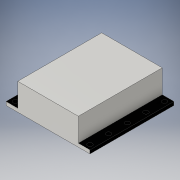
# Autodesk Inventor part: Legacy Module
Saved by Autodesk Inventor 2016 (Build 200138000, 138)
## iProperties
Created: 2016-01-08
Part Number: Legacy Module
Material: Generic
Document SubType Name: Modeling
Designer: TimB
Density: 1 g/cm^3
Appearance: Black
Author: TimB
Autodesk Inventor part; units mm, degrees
ref_plane "YZ Plane" through (0, 0, 0) normal (1, 0, 0) x (0, 1, 0)
ref_plane "XZ Plane" through (0, 0, 0) normal (0, 1, 0) x (-1, 0, 0)
ref_plane "XY Plane" through (0, 0, 0) normal (0, 0, 1) x (1, 0, 0)
sketch "Sketch1" plane through (0, 0, 0) normal (0, 1, 0) x (-1, 0, 0)
  line L0 (-36, -36) -> (36, -36)
  line L1 (36, -36) -> (36, 36)
  line L2 (36, 36) -> (-36, 36)
  line L3 (-36, 36) -> (-36, -36)
  line L4 (-36, -36) -> (36, 36) construction
  line L5 (36, -36) -> (-36, 36) construction
  point P0 (0, 0)
  dimension "d0" = 72
  dimension "d1" = 72
  constraints: 12 end point, 2 midpoint, 2 parallel, 1 horizontal, 1 perpendicular
  measures "d0" distance of L2.end L1.end
  measures "d1" distance of L1.end L0.end
extrude "Extrusion1" add sketch "Sketch1" along normal blind 3
sketch "Sketch2" plane through (0, 3, 0) normal (0, 1, 0) x (1, 0, 0)
  line L0 (-36, -36) -> (36, -36) projected
  line L1 (26, 36) -> (-26, 36)
  line L2 (-26, 36) -> (-26, -36)
  line L3 (-26, -36) -> (26, -36)
  line L4 (26, -36) -> (26, 36)
  line L5 (26, 36) -> (-26, -36) construction
  line L6 (-26, 36) -> (26, -36) construction
  point P0 (0, 0)
  dimension "d4" = 52
  constraints: 12 end point, 2 midpoint, 2 parallel, 1 horizontal, 1 perpendicular, 1 point on line
  measures "d4" distance of L3.end L2.end
extrude "Extrusion2" add sketch "Sketch2" along normal blind 20
sketch "Sketch3" plane through (0, 0, 0) normal (0, -1, 0) x (1, 0, 0)
  line L0 (-36, 36) -> (36, 36) projected
  line L1 (-36, 36) -> (-32, 36)
  line L2 (-32, 36) -> (-32, 32)
  line L3 (-32, 32) -> (-36, 32)
  line L4 (-36, 32) -> (-36, 36)
  circle A0 centre (-32, 16) radius 1.85 projected
  circle A1 centre (-32, 0) radius 1.85 projected
  circle A2 centre (-32, -16) radius 1.85 projected
  circle A3 centre (-32, -32) radius 1.85 projected
  point P0 (0, 0)
  dimension "d7" = 4
  dimension "d8" = 4
  constraints: 8 end point, 2 parallel, 1 horizontal, 1 perpendicular
  measures "d7" distance of L2.end L3.end
  measures "d8" distance of L1.end L2.end
hole "Hole2" at (-32, 0, 32) at (-32, 0, 16) at (-32, 0, 0) at (-32, 0, -16) at (-32, 0, -32) direction (0, 1, 0) diameter 4 end through all
sketch "Sketch4" plane through (0, 0, 0) normal (0, -1, 0) x (1, 0, 0)
  circle A0 centre (32, -32) radius 1.85 projected
  circle A1 centre (32, -16) radius 1.85 projected
  circle A2 centre (32, 0) radius 1.85 projected
  circle A3 centre (32, 16) radius 1.85 projected
  circle A4 centre (32, 32) radius 1.85 projected
  point P0 (0, 0)
hole "Hole4" at (32, 0, 32) at (32, 0, 16) at (32, 0, 0) at (32, 0, -16) at (32, 0, -32) direction (0, 1, 0) diameter 4 end through all
body "Solid1"
